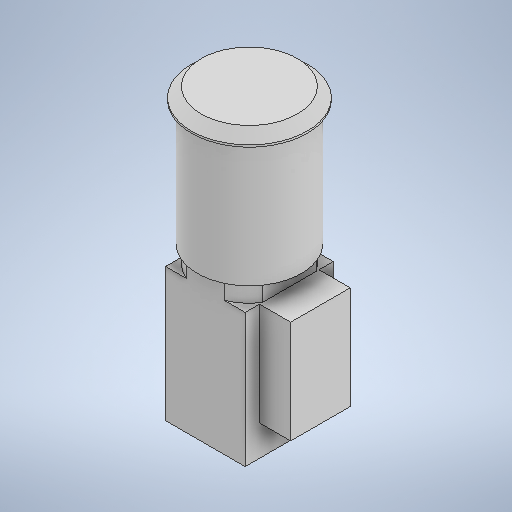
# Autodesk Inventor part: LEDpower_switch
Saved by Autodesk Inventor 2025.1 (Build 291241000, 241)
## iProperties
Created: 2026-04-16
Part Number: LEDpower_switch
Material: Generic
Document SubType Name: Modeling
Designer: User
Density: 1 g/cm^3
Appearance: Default
Author: User
Autodesk Inventor part; units mm, degrees
ref_plane "YZ Plane" through (0, 0, 0) normal (1, 0, 0) x (0, 1, 0)
ref_plane "XZ Plane" through (0, 0, 0) normal (0, 1, 0) x (-1, 0, 0)
ref_plane "XY Plane" through (0, 0, 0) normal (0, 0, 1) x (1, 0, 0)
sketch "Sketch1" plane through (0, 0, 0) normal (0, 1, 0) x (-1, 0, 0)
  circle A0 centre (0, 0) radius 7.9
  dimension "d0" = 15.8
  constraints: 1 centre point, 1 coincident
  measures "d0" diameter of A0
extrude "Extrusion1" add sketch "Sketch1" along normal blind 18.9
sketch "Sketch2" plane through (0, 18.9, 0) normal (0, 1, 0) x (1, 0, 0)
  circle A0 centre (0, 0) radius 8.8
  dimension "d3" = 17.6
  constraints: 1 centre point, 1 coincident
  measures "d3" diameter of A0
extrude "Extrusion2" add sketch "Sketch2" along normal blind 1.8
chamfer "Chamfer1" distance 1.5 angle 45 1 edges at (-8.8, 20.7, 0)
sketch "Sketch3" plane through (0, 0, 0) normal (0, -1, 0) x (1, 0, 0)
  line L0 (6.05, 6.7) -> (-6.05, 6.7)
  line L1 (-6.05, 6.7) -> (-6.05, -6.7)
  line L2 (-6.05, -6.7) -> (6.05, -6.7)
  line L3 (6.05, -6.7) -> (6.05, 6.7)
  line L4 (6.05, 6.7) -> (-6.05, -6.7) construction
  line L5 (-6.05, 6.7) -> (6.05, -6.7) construction
  point P0 (0, 0)
  dimension "d9" = 12.1
  dimension "d10" = 13.4
  constraints: 12 end point, 2 midpoint, 2 parallel, 1 horizontal, 1 perpendicular
  measures "d9" distance of L2.end L1.end
  measures "d10" distance of L1.end L0.end
extrude "Extrusion3" add sketch "Sketch3" along normal blind 23
sketch "Sketch4" plane through (0, -23, 0) normal (0, -1, 0) x (1, 0, 0)
  line L0 (6.05, -6.7) -> (6.05, 6.7) projected
  line L1 (10.8, 4.525) -> (1.3, 4.525)
  line L2 (1.3, 4.525) -> (1.3, -4.525)
  line L3 (1.3, -4.525) -> (10.8, -4.525)
  line L4 (10.8, -4.525) -> (10.8, 4.525)
  line L5 (6.05, 5.0801) -> (6.05, -5.0801) projected
  line L6 (10.8, 4.525) -> (1.3, -4.525) construction
  line L7 (1.3, 4.525) -> (10.8, -4.525) construction
  point P0 (0, 0)
  point P1 (6.05, 0)
  dimension "d13" = 9.5
  dimension "d14" = 9.05
  constraints: 12 end point, 3 midpoint, 2 parallel, 1 horizontal, 1 perpendicular
  measures "d13" distance of L3.end L2.end
  measures "d14" distance of L2.end L1.end
extrude "Extrusion4" add sketch "Sketch4" against normal blind 20.3
sketch "Sketch5" plane through (10.8, -23, 4.525) normal (1, 0, 0) x (0, 0, -1)
  line L0 (9.05, 0) -> (0, 0) projected
  line L1 (9.05, 4.67) -> (0, 4.67)
  line L2 (0, 4.67) -> (9.05, 4.67)
  line L3 (9.05, 4.67) -> (9.05, 0)
  line L4 (9.05, 0) -> (0, 0)
  line L5 (0, 0) -> (0, 4.67)
  point P0 (4.525, 23)
  point P1 (9.05, 4.67)
  dimension "d17" = 4.67
  constraints: 10 end point, 3 parallel, 1 horizontal, 1 perpendicular
  measures "d17" distance between parallel lines of L0 L1
extrude "Extrusion5" cut sketch "Sketch5" against normal up to surface (4.75 mm away)
sketch "Sketch6" plane through (0, 0, 0) normal (0, 1, 0) x (1, 0, 0)
  circle A0 centre (0, 0) radius 7.3 projected
  circle A1 centre (0, 0) radius 8.35
  line L0 (6.05, -6.7) -> (4.1857, -6.7) projected
  line L1 (-4.1857, -6.7) -> (4.1857, -6.7) projected
  line L2 (-4.1857, -6.7) -> (-6.05, -6.7) projected
  line L3 (6.05, -6.7) -> (-6.05, -6.7) projected
  line L4 (6.05, -4.525) -> (6.05, 4.525) projected
  line L5 (6.05, -4.525) -> (6.05, 4.525) projected
  line L6 (6.05, 6.7) -> (6.05, -6.7) projected
  line L7 (6.05, 6.7) -> (6.05, 5.0801) projected
  line L8 (6.05, -5.0801) -> (6.05, 5.0801) projected
  line L9 (6.05, -5.0801) -> (6.05, -6.7) projected
  line L10 (-6.05, 6.7) -> (-4.1857, 6.7) projected
  line L11 (4.1857, 6.7) -> (-4.1857, 6.7) projected
  line L12 (4.1857, 6.7) -> (6.05, 6.7) projected
  line L13 (-6.05, 6.7) -> (6.05, 6.7) projected
  line L14 (-6.05, -6.7) -> (-6.05, -5.0801) projected
  line L15 (-6.05, 5.0801) -> (-6.05, -5.0801) projected
  line L16 (-6.05, 5.0801) -> (-6.05, 6.7) projected
  line L17 (-6.05, -6.7) -> (-6.05, 6.7) projected
  point P0 (6.05, -5.755)
  point P1 (6.05, 5.755)
  point P2 (4.9832, 6.7)
  point P3 (-4.9832, 6.7)
  point P4 (-6.05, 5.755)
  point P5 (-6.05, -5.755)
  point P6 (-4.9832, -6.7)
  point P7 (4.9832, -6.7)
  dimension "d20" = 16.7
  constraints: 1 centre point, 1 coincident
  measures "d20" diameter of A1
extrude "Extrusion6" cut sketch "Sketch6" against normal up to surface (2.7 mm away) contours A0 L4 L6 A1 | A0 L11 L12 A1 L6 L4 | L4 L6 A1 L0 L1 A0 | A0 L11 L10 A1 L12 | L1 L0 A1 L2 A0 | A0 L15 L16 A1 L10 L11 | L1 L2 A1 L14 L15 A0 | A0 L15 L14 A1 L16 | L12 L6 A1 | A1 L6 L0 | A1 L16 L10 | L2 L14 A1
body "Solid1"
